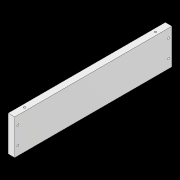
# Autodesk Inventor part: AfterComp1Chassis
Saved by Autodesk Inventor 2021 (Build 250183000, 183)
## iProperties
Created: 2021-02-15
Part Number: AfterComp1Chassis
Material: UHMW, White
Document SubType Name: Modeling
Designer: Esketitttttt
Density: 0.94 g/cm^3
Appearance: Smooth - White
Mass: 46.3515 g
Surface Area: 256.262 cm^2
Volume: 49.3101 cm^3
Author: Esketitttttt
Autodesk Inventor part; units mm, degrees
ref_plane "YZ Plane" through (0, 0, 0) normal (1, 0, 0) x (0, 1, 0)
ref_plane "XZ Plane" through (0, 0, 0) normal (0, 1, 0) x (-1, 0, 0)
sketch "BasePlan" plane through (0, 0, 0) normal (0, 1, 0) x (-1, 0, 0)
  line L0 (0, 0) -> (-35.15, 0)
  line L1 (-35.15, 0) -> (-35.15, -20.254)
  line L2 (-35.15, -20.254) -> (0, -20.254)
  line L3 (0, -20.254) -> (0, 0)
  line L4 (0, 0) -> (-16.1, 0)
  line L5 (-16.1, 0) -> (-16.1, 41.82)
  line L6 (-16.1, 41.82) -> (0, 41.82)
  line L7 (0, 41.82) -> (0, 0)
  line L8 (-16.1, 41.82) -> (-35.15, 41.82)
  line L9 (-35.15, 41.82) -> (-35.15, 0)
  line L10 (-35.15, 0) -> (-16.1, 0)
  line L11 (-16.1, 0) -> (-16.1, 41.82)
  line L12 (0, 0) -> (0, -10.127)
  line L13 (0, -10.127) -> (8.9825, -10.127) construction
  line L14 (-16.1, -20.254) -> (-16.1, -62.074)
  line L15 (-16.1, -62.074) -> (0, -62.074)
  line L16 (0, -62.074) -> (0, -20.254)
  line L17 (-16.1, -62.074) -> (-35.15, -62.074)
  line L18 (-35.15, -62.074) -> (-35.15, -20.254)
  line L19 (0, -62.074) -> (4.7625, -62.074) construction
  line L20 (4.7625, -62.074) -> (4.7625, -66.8365) construction
  line L21 (4.7625, -66.8365) -> (0, -66.8365) construction
  line L22 (0, -66.8365) -> (0, -62.074) construction
  line L23 (0, 41.82) -> (4.7625, 41.82) construction
  line L24 (4.7625, 41.82) -> (4.7625, 46.5825) construction
  line L25 (4.7625, 46.5825) -> (0, 46.5825) construction
  line L26 (0, 46.5825) -> (0, 41.82) construction
  line L27 (-35.15, -62.074) -> (-39.9125, -62.074) construction
  line L28 (-39.9125, -62.074) -> (-39.9125, -66.8365) construction
  line L29 (-39.9125, -66.8365) -> (-35.15, -66.8365) construction
  line L30 (-35.15, -66.8365) -> (-35.15, -62.074) construction
  line L31 (-35.15, 41.82) -> (-39.9125, 41.82) construction
  line L32 (-39.9125, 41.82) -> (-39.9125, 46.5825) construction
  line L33 (-39.9125, 46.5825) -> (-35.15, 46.5825) construction
  line L34 (-35.15, 46.5825) -> (-35.15, 41.82) construction
  line L35 (-39.9125, 46.5825) -> (-35.15, 46.5825)
  line L36 (-35.15, 46.5825) -> (-35.15, 0)
  line L37 (-35.15, 0) -> (-39.9125, 0)
  line L38 (-39.9125, 0) -> (-39.9125, 46.5825)
  line L39 (4.7625, 46.5825) -> (0, 46.5825)
  line L40 (0, 46.5825) -> (0, -66.8365)
  line L41 (0, -66.8365) -> (4.7625, -66.8365)
  line L42 (4.7625, -66.8365) -> (4.7625, 46.5825)
  line L43 (-35.15, 46.5825) -> (0, 46.5825)
  line L44 (0, 46.5825) -> (0, 41.82)
  line L45 (0, 41.82) -> (-35.15, 41.82)
  line L46 (-35.15, 41.82) -> (-35.15, 46.5825)
  line L47 (-35.15, -62.074) -> (0, -62.074)
  line L48 (0, -62.074) -> (0, -66.8365)
  line L49 (0, -66.8365) -> (-35.15, -66.8365)
  line L50 (-35.15, -66.8365) -> (-35.15, -62.074)
  line L51 (-39.9125, -66.8365) -> (-35.15, -66.8365)
  line L52 (-35.15, -66.8365) -> (-35.15, -20.254)
  line L53 (-35.15, -20.254) -> (-39.9125, -20.254)
  line L54 (-39.9125, -20.254) -> (-39.9125, -66.8365)
  point P0 (0, -62.074)
  point P1 (-35.15, 0)
  dimension "d3" = 16.1
  dimension "d5" = 19.05
  dimension "d6" = 20.254
  dimension "d7" = 41.82
  dimension "d8" = 35.15
  dimension "d9" = 35.15
  dimension "d10" = 10.127
  dimension "d12" = 4.7625
  constraints: 110 end point, 24 parallel, 13 horizontal, 12 perpendicular, 7 equal length, 5 symmetric about line, 1 midpoint, 1 point on line
  measures "d3" distance of L5.end L6.end
  measures "d5" distance of L5.end L8.end
  measures "d6" distance of L2.end L0.start
  measures "d7" distance of L6.end L0.start
  measures "d8" distance of L8.end L6.end
  measures "d9" distance of L1.end L2.end
  measures "d10" distance of L0.start L12.end
  measures "d12" distance of L19.end L20.end
extrude "BackWall" add sketch "BasePlan" along normal blind 25.4 contours L7 L40 L39 L42 L41 L16 L3
sketch "Sketch2" plane through (-4.7625, 0, -66.8365) normal (-1, 0, 0) x (0, 0, 1)
  line L0 (0, 0) -> (0, 25.4) construction
  line L1 (0, 0) -> (113.419, 0) construction
  line L2 (0, 0) -> (2.3812, 0) construction
  line L3 (2.3812, 0) -> (2.3812, 6.35) construction
  line L4 (2.3812, 6.35) -> (0, 6.35) construction
  line L5 (0, 6.35) -> (0, 0) construction
  line L6 (2.3812, 0) -> (2.3812, 19.05) construction
  line L7 (0, 25.4) -> (113.419, 25.4) projected
  line L8 (0, 25.4) -> (56.7095, 25.4) construction
  line L9 (56.7095, 25.4) -> (56.7095, 53.975) construction
  point P0 (66.8365, 0)
  point P1 (4.7625, 0)
  point P2 (111.0377, 19.05)
  point P3 (111.0378, 6.35)
  dimension "d25" = 4.7625
  dimension "d26" = 25.4
  dimension "d27" = 2.3813
  dimension "d28" = 6.35
  dimension "d29" = 19.05
  dimension "d30" = 113.419
  dimension "d31" = 56.7095
  constraints: 14 end point, 2 coincident, 2 parallel, 2 symmetric about line, 1 horizontal, 1 midpoint, 1 perpendicular, 1 point on line, 1 vertical
  measures "d25" distance of L0.start point (4.763, 0)
  measures "d26" distance of L0.start L0.end
  measures "d27" distance of L4.end L3.end
  measures "d28" distance of L3.end L2.end
  measures "d29" distance of L2.end L6.end
  measures "d30" distance of L0.end L7.end
  measures "d31" distance of L0.end L8.end
extrude "LeftSideWall" [suppressed]
extrude "RightSideWall" [suppressed]
hole "BackHoles" at (-4.7625, 6.35, -64.4553) at (-4.7625, 19.05, -64.4553) at (-4.7625, 19.05, 44.2012) at (-4.7625, 6.35, 44.2013) direction (1, 0, 0) diameter 1.524 depth 9.525 tip angle 118
extrude "RightFrontWall" [suppressed]
extrude "LeftFrontWall" [suppressed]
sketch "Sketch3" plane through (39.9125, 0, 46.5825) normal (1, 0, 0) x (0, 0, -1)
  line L0 (0, 0) -> (2.3812, 0) construction
  line L1 (2.3812, 0) -> (2.3812, 6.35) construction
  line L2 (2.3812, 6.35) -> (0, 6.35) construction
  line L3 (0, 6.35) -> (0, 0) construction
  line L4 (2.3812, 0) -> (2.3812, 19.05) construction
  line L5 (0, 25.4) -> (57.8525, 25.4) construction
  line L6 (57.8525, 25.4) -> (57.8525, 53.975) construction
  point P0 (69.1225, 0)
  point P1 (4.7625, 0)
  point P2 (115.705, 25.4)
  point P3 (113.3237, 19.05)
  point P4 (113.3238, 6.35)
  dimension "d39" = 4.7625
  dimension "d40" = 25.4
  dimension "d41" = 2.3813
  dimension "d42" = 6.35
  dimension "d43" = 19.05
  dimension "d44" = 115.705
  dimension "d45" = 57.8525
  constraints: 14 end point, 2 coincident, 2 parallel, 2 symmetric about line, 1 horizontal, 1 perpendicular, 1 point on line, 1 vertical
  measures "d39" distance of L0.start point (4.763, 0)
  measures "d40" distance of L0.start L5.start
  measures "d41" distance of L2.end L1.end
  measures "d42" distance of L1.end L0.end
  measures "d43" distance of L0.end L4.end
  measures "d44" distance of L5.start point (115.705, 25.4)
  measures "d45" distance of L5.start L5.end
hole "FrontHoles" [suppressed]
ref_plane "Work Plane1" through (0, -3.175, 0) normal (0, -1, 0) x (1, 0, 0)
sketch "Sketch4" plane through (0, -3.175, 0) normal (0, -1, 0) x (1, 0, 0)
  line L0 (-4.7625, 43.4392) -> (-4.7625, 44.9632) projected
  line L1 (-4.7625, 43.4393) -> (-4.7625, 44.9633) projected
  line L2 (-4.7625, -65.2173) -> (-4.7625, -63.6933) construction
  line L3 (-4.7625, -65.2173) -> (-4.7625, -63.6933) construction
  line L4 (-4.7625, -66.8365) -> (-4.7625, 46.5825) projected
  line L5 (-4.7625, 46.5825) -> (0, 46.5825) projected
  line L6 (0, 46.5825) -> (0, -66.8365) projected
  line L7 (0, -66.8365) -> (-4.7625, -66.8365) projected
  line L8 (-4.7625, -66.8365) -> (0, -66.8365) construction
  line L9 (0, -64.36) -> (-3.9052, -64.36) construction
  line L10 (-2.3813, -64.36) -> (-2.3813, -57.3115) construction
  line L11 (0, 46.5825) -> (0, -66.8365) projected
  line L12 (0, -10.127) -> (-4.7625, -10.127)
  point P0 (0, 0)
  point P1 (-2.3813, 37.0575)
  dimension "d55" = 7.0485
  dimension "d74" = 2.3813
  constraints: 8 end point, 2 midpoint, 1 coincident, 1 horizontal, 1 parallel, 1 symmetric about line
  measures "d55" distance of L10.end L10.start
  measures "d74" distance from line of L4 L10.end
hole "BottomHoles" at (-2.3813, -3.175, -57.3115) at (-2.3813, -3.175, 37.0575) direction (0, 1, 0) diameter 1.524 depth 9.525 tip angle 118
sketch "Sketch5" plane through (0, 25.4, 0) normal (0, 1, 0) x (1, 0, 0)
  line L0 (-4.7625, -46.5825) -> (0, -46.5825) construction
  line L1 (0, -46.5825) -> (0, -41.82) construction
  line L2 (0, -41.82) -> (-4.7625, -41.82) construction
  line L3 (-4.7625, -41.82) -> (-4.7625, -46.5825) construction
  line L4 (-4.7625, -41.82) -> (-2.3812, -41.82) construction
  line L5 (-2.3812, -41.82) -> (-2.3812, -37.0575) construction
  line L6 (-2.3812, -37.0575) -> (-4.7625, -37.0575) construction
  line L7 (-4.7625, -37.0575) -> (-4.7625, -41.82) construction
  line L8 (17.575, -64.36) -> (17.575, -69.1225)
  line L9 (20.7687, 10.127) -> (-4.7625, 10.127)
  line L10 (-4.7625, -46.5825) -> (0, -46.5825) projected
  line L11 (-4.7625, 66.8365) -> (-4.7625, -46.5825) projected
  line L12 (-4.7625, 10.127) -> (-15.875, 10.127)
  point P0 (0, 0)
  point P1 (-2.3812, 57.3115)
  point P2 (-2.3812, 57.3115)
  point P3 (37.5312, -37.0575)
  point P4 (37.5312, -37.0575)
  point P5 (37.5312, 57.3115)
  point P6 (37.5312, 57.3115)
  point P7 (39.9125, -46.5825)
  dimension "d63" = 17.7775
  dimension "d64" = 2.3813
  dimension "d65" = 4.7625
  dimension "d66" = 0
  constraints: 22 end point, 6 symmetric about line, 4 parallel, 3 horizontal, 2 coincident, 2 perpendicular, 1 midpoint
  measures "d64" distance of L6.end L5.end
  measures "d65" distance of L5.end L4.end
  measures "d66" distance between parallel lines of L12 L9
hole "TopHoles" at (-2.3812, 25.4, 37.0575) at (-2.3812, 25.4, -57.3115) at (37.5312, 25.4, 37.0575) at (37.5312, 25.4, -57.3115) direction (0, -1, 0) diameter 1.524 depth 6.35 tip angle 118
equation "\"d9\" = d8"
equation "\"d10\" = 0.5 * d6"
equation "\"d27\" = 0.5 * d25"
equation "\"d28\" = 0.25 * d26"
equation "\"d29\" = 3 * d28"
equation "\"d31\" = 0.5 * d30"
equation "\"d41\" = 0.5 * d39"
equation "\"d42\" = 0.25 * d40"
equation "\"d43\" = 3 * d42"
equation "\"d45\" = 0.5 * d44"
body "Solid1"
